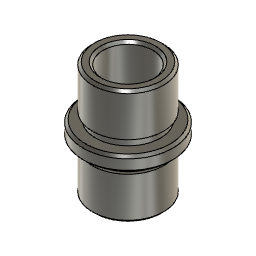
Model 1 (Autodesk Fusion 360 design; units mm, degrees)
Autodesk Fusion 360 part; units mm, degrees
note: some values were not read from the file. Chosen so that the rebuilt part matches the saved one: which face or edge a step refers to; which pieces of a blend or face edit are solid. Set by a fixed rule: which sketch regions a step uses.
sketch "Sketch1" plane through (0, 0, 0) normal (0, 0, 1) x (1, 0, 0)
  circle A0 centre (0, 0) radius 14.25
  dimension "d1" = 28.5
  constraint coincident A0.centre origin
  measures "d1" diameter of A0
extrude "Extrude1" add sketch "Sketch1" along normal blind 17 makes body 1
sketch "Sketch2" plane through (0, 0, 17) normal (0, 0, 1) x (-1, 0, 0)
  circle A0 centre (0, 0) radius 14.25
  circle A1 centre (0, 0) radius 13
  dimension "d4" = 26
  constraint coincident A0.centre A1.centre
  measures "d4" diameter of A1
extrude "Extrude2" add sketch "Sketch2" along normal blind 3 separate body contours A1 makes body 2
sketch "Sketch3" plane through (0, 0, 20) normal (0, 0, 1) x (-1, 0, 0)
  circle A0 centre (0, 0) radius 13
  circle A1 centre (0, 0) radius 18
  dimension "d7" = 36
  constraint coincident A0.centre A1.centre
  measures "d7" diameter of A1
extrude "Extrude3" add sketch "Sketch3" along normal blind 6 separate body makes body 3
move_face "OffsetFaces2" offset 10 1 faces at (-12.9838, 0.648, 24) on bodies 3
sketch "Sketch4" plane through (0, 0, 26) normal (0, 0, 1) x (-1, 0, 0)
  circle A0 centre (0, 0) radius 18
  circle A1 centre (0, 0) radius 13
  circle A2 centre (0, 0) radius 3
  dimension "d10" = 26
  constraint coincident A0.centre A1.centre
  measures "d10" diameter of A1
extrude "Extrude5" add sketch "Sketch4" along normal blind 3 separate body contours A1 | A2 makes body 4
sketch "Sketch5" plane through (0, 0, 29) normal (0, 0, 1) x (-1, 0, 0)
  circle A0 centre (0, 0) radius 13
  circle A1 centre (0, 0) radius 14.25
  dimension "d15" = 28.5
  measures "d15" diameter of A1
extrude "Extrude6" add sketch "Sketch5" along normal blind 17 separate body makes body 5
move_face "OffsetFaces3" offset 13 1 faces at (-12.9838, 0.648, 40.3333) on bodies 5
sketch "Sketch6" plane through (0, 0, 46) normal (0, 0, 1) x (-1, 0, 0)
  circle A0 centre (0, 0) radius 14.25
  circle A1 centre (0, 0) radius 10
  dimension "d21" = 20
  constraint coincident A0.centre A1.centre
  measures "d21" diameter of A1
extrude "Extrude7" cut sketch "Sketch6" against normal blind 46 contours A1 bodies 1 2 3 4 5
chamfer "Chamfer1" distance 1 angle 45 1 faces at (-12.743, 1.2048, 46) on bodies 5
chamfer "Chamfer2" distance 1 angle 45 1 faces at (-15.2663, -0.8943, 26) on bodies 3
chamfer "Chamfer3" distance 1 angle 45 1 faces at (-15.2663, -0.8943, 20) on bodies 3
chamfer "Chamfer4" distance 1 angle 45 1 faces at (12.743, -1.2048, 0) on bodies 1
